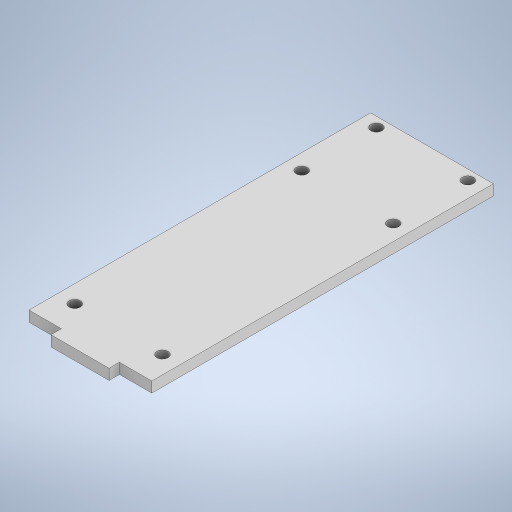
# Autodesk Inventor part: Basis of the robot
Saved by Autodesk Inventor 2023 (Build 270158000, 158)
## iProperties
Created: 2023-05-15
Part Number: Basis of the robot
Material: Типовые
Document SubType Name: Modeling
Designer: ivanc
Density: 1 g/cm^3
Appearance: По умолчанию
Author: ivanc
Autodesk Inventor part; units mm, degrees
ref_plane "YZ Plane" through (0, 0, 0) normal (1, 0, 0) x (0, 1, 0)
ref_plane "XZ Plane" through (0, 0, 0) normal (0, 1, 0) x (-1, 0, 0)
ref_plane "XY Plane" through (0, 0, 0) normal (0, 0, 1) x (1, 0, 0)
sketch "Эскиз1" plane through (0, 0, 0) normal (0, 1, 0) x (-1, 0, 0)
  line L0 (-8.725, 50) -> (8.725, 50)
  line L1 (8.725, 50) -> (8.725, -50)
  line L2 (8.725, -50) -> (-8.725, -50)
  line L3 (-8.725, -50) -> (-8.725, 50)
  line L4 (-8.725, 50) -> (8.725, -50) construction
  line L5 (8.725, 50) -> (-8.725, -50) construction
  line L6 (-8.725, 50) -> (0.475, 50)
  line L7 (0.475, 50) -> (0.475, 47.05)
  line L8 (0.475, 47.05) -> (-8.725, 47.05)
  line L9 (-8.725, 47.05) -> (-8.725, 50)
  point P0 (0, 0)
  point P1 (0.475, 50)
  dimension "d0" = 17.45
  dimension "d1" = 100
  dimension "d13" = 9.2
  dimension "d14" = 2.95
  constraints: 20 end point, 4 parallel, 2 horizontal, 2 midpoint, 2 perpendicular
  measures "d0" distance of L1.end L2.end
  measures "d1" distance of L0.end L1.end
  measures "d13" distance of L7.end L8.end
  measures "d14" distance of L6.end L7.end
extrude "Выдавливание1" add sketch "Эскиз1" along normal blind 3 contours L0 L1 L2 L3 L8 L7
mirror "Зеркальное отражение1" about plane through (-8.725, 0, -50) normal (-1, 0, 0)
sketch "Эскиз2" plane through (0, 3, 0) normal (0, 1, 0) x (1, 0, 0)
  line L0 (-8.725, -50) -> (-8.725, -39.05) construction
  line L1 (-21.175, -39.05) -> (3.725, -39.05)
  line L2 (-0.475, -50) -> (-16.975, -50) projected
  line L3 (-21.725, 47.2) -> (4.275, 47.2)
  line L4 (-21.725, 26) -> (4.275, 26)
  line L5 (-8.725, 26) -> (-8.725, 47.2)
  line L6 (-8.725, 47.2) -> (-8.725, 50)
  line L7 (8.725, 50) -> (-26.175, 50) projected
  dimension "d4" = 10.95
  dimension "d5" = 24.9
  dimension "d15" = 26
  dimension "d16" = 2.8
  dimension "d17" = 21.2
  constraints: 12 end point, 5 midpoint, 3 horizontal, 2 perpendicular, 1 parallel, 1 vertical
  measures "d4" distance of L0.end L0.start
  measures "d5" distance of L1.start L1.end
  measures "d15" distance of L4.start L4.end
  measures "d16" distance of L5.end L6.end
  measures "d17" distance of L5.start L5.end
hole "Отверстие1" at (3.725, 3, 39.05) at (-21.175, 3, 39.05) at (-21.725, 3, -26) at (4.275, 3, -26) at (4.275, 3, -47.2) at (-21.725, 3, -47.2) direction (0, -1, 0) diameter 3.2 end through all
